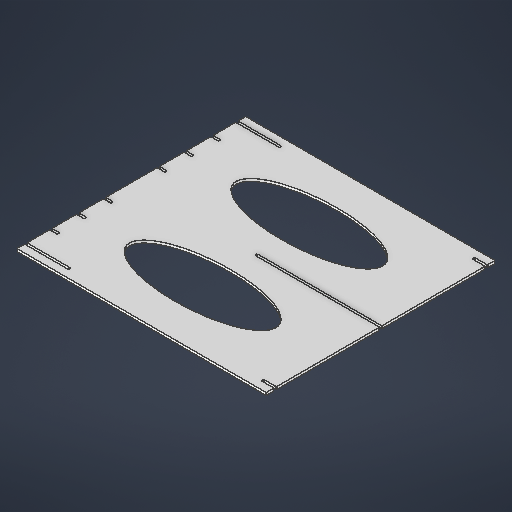
# Autodesk Inventor part: inside_leg
Saved by Autodesk Inventor 2027.1 (Build 311270010, 270A)
## iProperties
Created: 2025-09-11
Part Number: inside_leg
Material: Foam Core Board
Document SubType Name: Modeling
Designer: Nick
Density: 0.141998 g/cm^3
Appearance: Default(1)
Mass: 117.299 g
Surface Area: 3516.32 cm^2
Volume: 826.063 cm^3
Author: Nick
Autodesk Inventor part; units mm, degrees
ref_plane "YZ Plane" through (0, 0, 0) normal (1, 0, 0) x (0, 1, 0)
ref_plane "XZ Plane" through (0, 0, 0) normal (0, 1, 0) x (-1, 0, 0)
ref_plane "XY Plane" through (0, 0, 0) normal (0, 0, 1) x (1, 0, 0)
sketch "Sketch1" plane through (0, 0, 0) normal (0, 1, 0) x (-1, 0, 0)
  line L0 (0, 0) -> (485, 0)
  line L1 (485, 0) -> (485, -415)
  line L2 (485, -415) -> (0, -415)
  line L3 (0, -415) -> (0, 0)
  line L4 (485, -207.5) -> (0, -207.5)
  line L5 (0, -207.5) -> (0, 0)
  line L6 (0, -103.75) -> (100, -103.75)
  line L7 (485, -103.75) -> (385, -103.75)
  line L8 (242.5, 0) -> (242.5, -103.75)
  line L9 (242.5, -207.5) -> (242.5, -157.5)
  ellipse E0 centre (242.5, -103.75) end of major axis (385, -103.75) minor radius 53.75
  ellipse E1 centre (242.5, -311.25) end of major axis (385, -311.25) minor radius 53.75
  dimension "d0" = 485
  dimension "d1" = 415
  dimension "d2" = 100
  dimension "d3" = 100
  dimension "d4" = 103.75
  dimension "d5" = 50
  dimension "d6" = 103.75
  dimension "d7" = 103.75
  constraints: 20 end point, 5 midpoint, 2 horizontal, 2 parallel, 2 point on line, 2 vertical, 1 centre point, 1 coincident, 1 collinear, 1 perpendicular, 1 symmetric about line, 5 other
  measures "d0" distance of L1.end L2.end
  measures "d1" distance of L0.end L1.end
  measures "d2" distance of L6.start L6.end
  measures "d3" distance of L7.start L7.end
  measures "d4" distance between parallel lines of L0 L7
  measures "d5" distance of L9.start L9.end
  measures "d6" distance from line of L0 L6.end
  measures "d7" distance from line of L4 point (242.5, -103.75)
extrude "Extrusion1" add sketch "Sketch1" along normal blind 5 contours L0 L8 E0 L6 L3 | L0 L1 L7 E0 L8 | L6 E0 L9 L4 L3 | L4 L1 L2 L3 | L1 L4 L9 E0 L7
sketch "Sketch2" plane through (0, 5, 0) normal (0, 1, 0) x (1, 0, 0)
  line L0 (0, 0) -> (0, 415) projected
  line L1 (0, 207.5) -> (0, 209.75)
  line L2 (0, 209.75) -> (0, 207.5)
  line L3 (-485, 0) -> (0, 0) projected
  line L4 (-242.5, 0) -> (-242.5, 207.5)
  line L5 (0, 209.75) -> (-242.5, 209.75)
  line L6 (-242.5, 209.75) -> (-242.5, 205.25)
  line L7 (-242.5, 205.25) -> (0, 205.25)
  line L8 (0, 205.25) -> (0, 209.75)
  point P0 (0, 205.25)
  dimension "d10" = 2.25
  dimension "d11" = 4.5
  constraints: 14 end point, 2 midpoint, 2 parallel, 2 point on line, 1 collinear, 1 horizontal, 1 perpendicular, 1 vertical
  measures "d10" distance of L1.start L1.end
  measures "d11" distance of L6.end L5.end
extrude "Extrusion2" cut sketch "Sketch2" against normal blind 5 contours L7 L4 L6 L5 L0
sketch "Sketch3" plane through (-485, 0, 0) normal (0, 0, 1) x (1, 0, 0)
  line L0 (485, 0) -> (0, 0) projected
  line L1 (485, 0) -> (485, 5) projected
  line L2 (0, 0) -> (485, 0)
  line L3 (485, 0) -> (485, 5)
  line L4 (485, 5) -> (0, 5)
  line L5 (0, 5) -> (0, 0)
  constraints: 8 end point, 2 parallel, 1 horizontal, 1 perpendicular
extrude "Extrusion3" add sketch "Sketch3" along normal blind 15
sketch "Sketch4" plane through (0, 0, -415) normal (0, 0, -1) x (-1, 0, 0)
  line L0 (485, 0) -> (485, 5) projected
  line L1 (485, 5) -> (0, 5)
  line L2 (0, 5) -> (0, 0)
  line L3 (0, 0) -> (485, 0)
  line L4 (485, 0) -> (485, 5)
  constraints: 8 end point, 2 parallel, 1 horizontal, 1 perpendicular
extrude "Extrusion4" add sketch "Sketch4" along normal blind 15
sketch "Sketch5" plane through (0, 5, 0) normal (0, 1, 0) x (1, 0, 0)
  line L0 (-485, -15) -> (-485, 430) projected
  line L1 (-485, 207.5) -> (54.8472, 207.5)
  line L2 (-485, 0) -> (-400, 0)
  line L3 (-400, 0) -> (-400, 4.5)
  line L4 (-400, 4.5) -> (-485, 4.5)
  line L5 (-485, 4.5) -> (-485, 0)
  line L6 (0, 0) -> (-25, 0)
  line L7 (-25, 0) -> (-25, 4.5)
  line L8 (-25, 4.5) -> (0, 4.5)
  line L9 (0, 4.5) -> (0, 0)
  line L10 (0, -15) -> (-485, -15) projected
  line L11 (-485, 415) -> (-400, 415)
  line L12 (-400, 415) -> (-400, 410.5)
  line L13 (-400, 410.5) -> (-485, 410.5)
  line L14 (-485, 410.5) -> (-485, 415)
  line L15 (0, 415) -> (-25, 415)
  line L16 (-25, 415) -> (-25, 410.5)
  line L17 (-25, 410.5) -> (0, 410.5)
  line L18 (0, 410.5) -> (0, 415)
  dimension "d18" = 85
  dimension "d19" = 4.5
  dimension "d20" = 25
  dimension "d21" = 4.5
  dimension "d22" = 15
  constraints: 34 end point, 8 symmetric about line, 4 parallel, 3 horizontal, 2 perpendicular, 1 midpoint, 1 point on line
  measures "d18" distance of L4.end L3.end
  measures "d19" distance of L3.end L2.end
  measures "d20" distance of L7.end L8.end
  measures "d21" distance of L6.end L7.end
  measures "d22" distance between parallel lines of L10 L2
extrude "Extrusion5" cut sketch "Sketch5" against normal blind 5
sketch "Sketch6" plane through (0, 5, 0) normal (0, 1, 0) x (1, 0, 0)
  line L0 (-485, 4.5) -> (-485, 410.5) projected
  line L1 (-485, 4.5) -> (-485, 48.5)
  line L2 (-485, 48.5) -> (-470, 48.5)
  line L3 (-470, 48.5) -> (-470, 53)
  line L4 (-470, 53) -> (-485, 53)
  line L5 (-485, 53) -> (-485, 48.5)
  line L6 (-485, 100.75) -> (-470, 100.75)
  line L7 (-470, 100.75) -> (-470, 105.25)
  line L8 (-470, 105.25) -> (-485, 105.25)
  line L9 (-485, 105.25) -> (-485, 100.75)
  line L10 (-485, 153) -> (-470, 153)
  line L11 (-470, 153) -> (-470, 157.5)
  line L12 (-470, 157.5) -> (-485, 157.5)
  line L13 (-485, 157.5) -> (-485, 153)
  line L14 (-485, 205.25) -> (-470, 205.25)
  line L15 (-470, 205.25) -> (-470, 209.75)
  line L16 (-470, 209.75) -> (-485, 209.75)
  line L17 (-485, 209.75) -> (-485, 205.25)
  line L18 (-485, 257.5) -> (-470, 257.5)
  line L19 (-470, 257.5) -> (-470, 262)
  line L20 (-470, 262) -> (-485, 262)
  line L21 (-485, 262) -> (-485, 257.5)
  line L22 (-485, 309.75) -> (-470, 309.75)
  line L23 (-470, 309.75) -> (-470, 314.25)
  line L24 (-470, 314.25) -> (-485, 314.25)
  line L25 (-485, 314.25) -> (-485, 309.75)
  line L26 (-485, 362) -> (-470, 362)
  line L27 (-470, 362) -> (-470, 366.5)
  line L28 (-470, 366.5) -> (-485, 366.5)
  line L29 (-485, 366.5) -> (-485, 362)
  point P0 (0, 0)
  dimension "d25" = 44
  dimension "d26" = 15
  dimension "d27" = 4.5
  dimension "d30" = 52.25
  constraints: 58 end point, 2 parallel, 1 horizontal, 1 perpendicular, 1 point on line, 1 vertical, 48 other
  measures "d25" distance of L0.start L1.end
  measures "d26" distance of L4.end L3.end
  measures "d27" distance of L3.end L2.end
  measures "d30" distance of L1.end L6.start
extrude "Extrusion6" cut sketch "Sketch6" against normal blind 5 contours L0 L28 L27 L26 | L0 L24 L23 L22 | L0 L20 L19 L18 | L0 L12 L11 L10 | L0 L8 L7 L6 | L0 L4 L3 L2
fillet "Fillet1" radius 1 48 edges at (-485, 2.5, -4.5) (-485, 2.5, 0) (-485, 2.5, 15) (-400, 2.5, 0) (-400, 2.5, -4.5) (-470, 2.5, -48.5) (-470, 2.5, -53) (-485, 2.5, -53) (-485, 2.5, -48.5) (-470, 2.5, -100.75) (-470, 2.5, -105.25) (-485, 2.5, -105.25) (-485, 2.5, -100.75) (-485, 2.5, -157.5) (-485, 2.5, -153) (-470, 2.5, -153) (-470, 2.5, -157.5) (-470, 2.5, -257.5) (-470, 2.5, -262) (-485, 2.5, -262) (-485, 2.5, -257.5) (-485, 2.5, -314.25) (-485, 2.5, -309.75) (-470, 2.5, -309.75) (-470, 2.5, -314.25) (-470, 2.5, -362) (-470, 2.5, -366.5) (-485, 2.5, -366.5) (-485, 2.5, -362) (-485, 2.5, -410.5) (-485, 2.5, -415) (-400, 2.5, -410.5) (-400, 2.5, -415) (-485, 2.5, -430) (0, 2.5, -430) (0, 2.5, -415) (0, 2.5, -410.5) (-25, 2.5, -415) (-25, 2.5, -410.5) (-242.5, 2.5, -209.75) (-242.5, 2.5, -205.25) (0, 2.5, -209.75) (0, 2.5, -205.25) (0, 2.5, -4.5) (0, 2.5, 0) (-25, 2.5, -4.5) (-25, 2.5, 0) (0, 2.5, 15)
body "Solid1"
